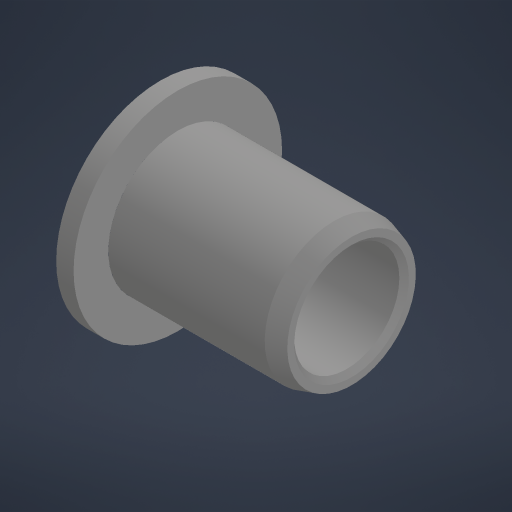
# Autodesk Inventor part: 80F-0610
Saved by Autodesk Inventor 2024.3 (Build 283343000, 343)
## iProperties
Created: 2024-01-24
Part Number: 80F-0610
Material: Generic
Catalog Web Link: www.cadenas.de
Description: Flange Bushings-80F
Vendor: OILES
Document SubType Name: Modeling
Designer: ASUS
Manufacturer: OILES
Mass: 0.211341 g
Surface Area: 4.76563 cm^2
Volume: 0.211341 cm^3
Density: 1 g/cm^3
Appearance: PSOLRGB-127-127-127
Category: PARTsolutions
Company: OILES
Title: 80F-0606
Author: Cadenas PARTsolutions
Comments: 80F
PSOL_IDENT_0: {$CADENAS_DATA/23d-libs/oiles/plastic_bearings/oiles_80/flange_bushings_80b.prj},166 {VTYP=3D},{NB=8
PSOL_IDENT_1: 0F-0606},{LINA=80F-0606},{NN=Flange Bushings},{DATE=15.04.2019 22:54:28},{GEOMDATE=07.11.2016 06:24:
PSOL_IDENT_2: 13},{VERSION=},{LINEID=190},{WBVAR=},{WBNUMERIC=}  {NB=80F-0606},{LINA=80F-0606},{KT=DUMMY},{ORDERNO=
PSOL_IDENT_3: 80F-0606},{S=6},{SRT=h7(0/-0.012)},{H=8},{HRT=H7(+0.015/0)},{ID=6},{IDT=+0.095/+0.045},{OD=8},{ODT=+
PSOL_IDENT_4: 0.157/+0.045},{F=12},{FT=1.0},{FTT=0/-0.10},{L=6},{LT=0/-0.3},{A=0.3},{B=1.0},{C=C0.3},{CC=0.300},{C
PSOL_IDENT_5: R=0.000},{TE=-40~80°C},{P=17.5N/mm2  (179kgf/cm2)},{V=0.85m/s  (51m/min)},{PV=2.45N/mm2•m/s  (1,500k
PSOL_IDENT_6: gf/cm2•m/min)},{AIT=The inner diameter tolerances are the values after pressing into a ring gauge of
PSOL_IDENT_7: OD+-0.002},{CAU=Please refer to catalog about detail.}
NB: 80F-0606
NN: Flange Bushings
NT: 80F
NBSYN: $ORDERNO.
LINA: 80F-0606
CATALOG: OILES CORPORATION
ORDERNO: 80F-0606
S: 6
SRT: h7(0/-0.012)
H: 8
HRT: H7(+0.015/0)
ID: 6
IDT: +0.095/+0.045
OD: 8
ODT: +0.157/+0.045
F: 12
FT: 1
FTT: 0/-0.10
L: 6
LT: 0/-0.3
TE: -40~80°C
P: 17.5N/mm2  (179kgf/cm2)
V: 0.85m/s  (51m/min)
PV: 2.45N/mm2•m/s  (1,500kgf/cm2•m/min)
AIT: The inner diameter tolerances are the values after pressing into a ring gauge of OD+-0.002.
CAU: Please refer to catalog about detail.
SUPPLIER: OILES
ARTICLENO: 80F-0606
BOMINFO: 80F-0606
CREATOR: CADENAS GmbH
Autodesk Inventor part; units mm, degrees
ref_plane "YZ Plane" through (0, 0, 0) normal (1, 0, 0) x (0, 1, 0)
ref_plane "XZ Plane" through (0, 0, 0) normal (0, 1, 0) x (-1, 0, 0)
ref_plane "XY Plane" through (0, 0, 0) normal (0, 0, 1) x (1, 0, 0)
sketch "Sketch_1" plane through (0, 0, 0) normal (0, 0, 1) x (1, 0, 0)
  line L0 (7, 0) -> (0, 0)
  line L1 (0, 3.3) -> (0.3, 3)
  line L2 (0.3, 3) -> (6.7, 3)
  line L3 (6.7, 3) -> (7, 3.3)
  line L4 (7, 3.3) -> (7, 3.7)
  line L5 (7, 3.7) -> (6, 4)
  line L6 (6, 4) -> (1, 4)
  line L7 (1, 4) -> (1, 6)
  line L8 (1, 6) -> (0, 6)
  line L9 (0, 6) -> (0, 3.3)
  constraints: 20 end point
revolve "Revolution1" add sketch "Sketch_1" angle 360 about axis through (7, 0, 0) along (1, 0, 0)
sketch "스케치2" plane through (0, 0, 0) normal (-1, 0, 0) x (0, 0, 1)
  circle A0 centre (0, 0) radius 3.3 projected
  circle A1 centre (0, 0) radius 6 projected
  circle A2 centre (0, 0) radius 3.025
  dimension "d1" = 6.05
  constraints: 1 centre point, 1 coincident
  measures "d1" diameter of A2
extrude "돌출1" cut sketch "스케치2" against normal up to surface (7 mm away) contours A2
move faces "이동1" translate (-2, 0, 0) faces at (0, 5.0099, -0.7419) (0.0917, 3.1979, -0.2582) (1, 5.2365, -0.7977) (0.6667, 5.9223, -0.9625)
move faces "이동2" translate (2, 0, 0) faces at (6.1667, -1.7292, 3.5514) (6.9083, 3.1979, -0.2582) (7, 3.5308, -0.2952)
body "Solid1"
